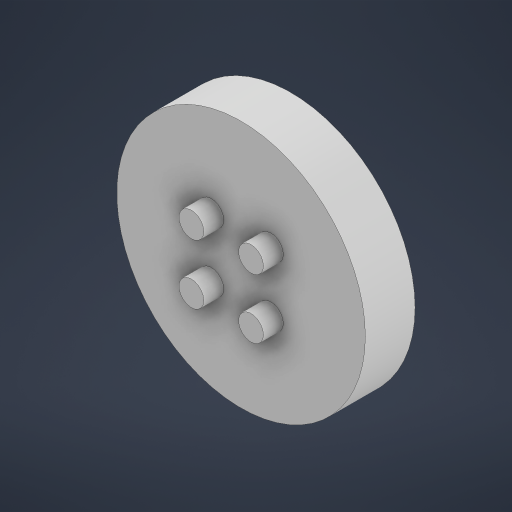
# Autodesk Inventor part: BaseH
Saved by Autodesk Inventor 2024 (Build 280153000, 153)
## iProperties
Created: 2023-05-12
Part Number: BaseH
Material: Genérico
Document SubType Name: Modeling
Designer: javie
Density: 1 g/cm^3
Appearance: Valor por defecto
Author: javie
Autodesk Inventor part; units mm, degrees
ref_plane "YZ Plane" through (0, 0, 0) normal (1, 0, 0) x (0, 1, 0)
ref_plane "XZ Plane" through (0, 0, 0) normal (0, 1, 0) x (-1, 0, 0)
ref_plane "XY Plane" through (0, 0, 0) normal (0, 0, 1) x (1, 0, 0)
sketch "Boceto1" plane through (0, 0, 0) normal (0, 0, 1) x (1, 0, 0)
  circle A0 centre (0, 0) radius 25
  dimension "d0" = 50
  constraints: 1 centre point, 1 coincident
  measures "d0" diameter of A0
extrude "Extrusión1" add sketch "Boceto1" along normal blind 10
sketch "Boceto3" plane through (0, 0, 10) normal (0, 0, 1) x (1, 0, 0)
  circle A0 centre (-6, -6) radius 2.5
  line L0 (0, 35) -> (0, -35) projected
  line L1 (-35, 0) -> (35, 0) projected
  circle A1 centre (6, -6) radius 2.5
  circle A2 centre (6, 6) radius 2.5
  circle A3 centre (-6, 6) radius 2.5
  line L2 (-18, -22) -> (18, -22)
  line L3 (18, -22) -> (18, 22)
  line L4 (18, 22) -> (-18, 22)
  line L5 (-18, 22) -> (-18, -22)
  point P0 (0, 0)
  dimension "d3" = 5
  dimension "d4" = 6
  dimension "d5" = 6
  dimension "d8" = 360
  dimension "d12" = 44
  dimension "d13" = 36
  dimension "d14" = 18
  dimension "d16" = 22
  constraints: 8 end point, 4 centre point, 2 parallel, 1 horizontal, 1 perpendicular, 9 other
  measures "d3" diameter of A0
  measures "d4" distance from line of L0 A0.centre
  measures "d5" distance from line of A0.centre L1
  measures "d12" distance of L4.end L2.start
  measures "d13" distance between parallel lines of L5 L3
  measures "d14" distance between parallel lines of L3 L0
  measures "d16" distance between parallel lines of L4 L1
extrude "Extrusión2" add sketch "Boceto3" along normal blind 4 contours A0 | A1 | A2 | A3
